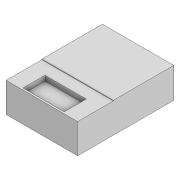
# Autodesk Inventor part: 00_HuaweiP30_Telelens
Saved by Autodesk Inventor 2022 (Build 260153000, 153)
## iProperties
Created: 2022-09-14
Part Number: 00_HuaweiP30_Telelens
Material: Generisch
Document SubType Name: Modeling
Designer: UC2
Density: 1 g/cm^3
Appearance: Vorgabe
Author: UC2
Autodesk Inventor part; units mm, degrees
ref_plane "YZ Plane" through (0, 0, 0) normal (1, 0, 0) x (0, 1, 0)
ref_plane "XZ Plane" through (0, 0, 0) normal (0, 1, 0) x (-1, 0, 0)
ref_plane "XY Plane" through (0, 0, 0) normal (0, 0, 1) x (1, 0, 0)
sketch "Skizze1" plane through (0, 0, 0) normal (0, 1, 0) x (-1, 0, 0)
  line L0 (-6.5, -8.75) -> (6.5, -8.75)
  line L1 (6.5, -8.75) -> (6.5, 8.75)
  line L2 (6.5, 8.75) -> (-6.5, 8.75)
  line L3 (-6.5, 8.75) -> (-6.5, -8.75)
  line L4 (-6.5, -8.75) -> (6.5, 8.75) construction
  line L5 (6.5, -8.75) -> (-6.5, 8.75) construction
  point P0 (0, 0)
  dimension "d0" = 13
  dimension "d1" = 17.5
  constraints: 12 end point, 2 midpoint, 2 parallel, 1 horizontal, 1 perpendicular
  measures "d0" distance of L2.end L1.end
  measures "d1" distance of L1.end L0.end
extrude "Extrusion1" add sketch "Skizze1" along normal blind 5.5
sketch "Skizze2" plane through (0, 5.5, 0) normal (0, 1, 0) x (1, 0, 0)
  line L0 (-6.5, 8.75) -> (-6.5, -8.75) projected
  line L1 (-6.5, -8.75) -> (6.5, -8.75) projected
  line L2 (6.5, -8.75) -> (6.5, 8.75) projected
  line L3 (6.5, 8.75) -> (-6.5, 8.75) projected
  line L4 (3.75, -4.4349) -> (-3.75, -4.4349)
  line L5 (-3.75, -4.4349) -> (-3.75, -8.4349)
  line L6 (-3.75, -8.4349) -> (3.75, -8.4349)
  line L7 (3.75, -8.4349) -> (3.75, -4.4349)
  line L8 (3.75, -4.4349) -> (-3.75, -8.4349) construction
  line L9 (-3.75, -4.4349) -> (3.75, -8.4349) construction
  point P0 (0, 0)
  point P1 (0, -6.4349)
  dimension "d4" = 7.5
  dimension "d5" = 4
  constraints: 12 end point, 2 midpoint, 2 parallel, 1 horizontal, 1 perpendicular
  measures "d4" distance of L6.end L5.end
  measures "d5" distance between parallel lines of L4 L6
extrude "Extrusion2" cut sketch "Skizze2" against normal blind 1 contours L7 L6 L5 L4
sketch "Skizze3" plane through (0, 5.5, 0) normal (0, 1, 0) x (1, 0, 0)
  line L0 (-6.5, 8.75) -> (-6.5, -8.75) projected
  line L1 (3.75, -8.4349) -> (-3.75, -8.4349) projected
  line L2 (-3.75, -8.4349) -> (-3.75, -4.4349) projected
  line L3 (-3.75, -4.4349) -> (3.75, -4.4349) projected
  line L4 (3.75, -4.4349) -> (3.75, -8.4349) projected
  line L5 (-6.5, 8.75) -> (-6.5, -8.75) projected
  line L6 (-6.5, -8.75) -> (6.5, -8.75) projected
  line L7 (6.5, -8.75) -> (6.5, 8.75) projected
  line L8 (6.5, 8.75) -> (-6.5, 8.75) projected
  line L9 (6.5, -8.75) -> (6.5, 8.75) projected
  line L10 (-6.5, -8.75) -> (6.5, -8.75)
  line L11 (6.5, -8.75) -> (6.5, -2.25)
  line L12 (6.5, -2.25) -> (-6.5, -2.25)
  line L13 (-6.5, -2.25) -> (-6.5, -8.75)
  point P0 (0, 0)
  dimension "d8" = 6.5
  constraints: 8 end point, 2 parallel, 1 horizontal, 1 perpendicular, 1 point on line
  measures "d8" distance of L11.end L10.end
extrude "Extrusion3" cut sketch "Skizze3" against normal blind 0.1 contours L12 L7 L6 L0
sketch "Skizze4" plane through (6.5, 0, -8.75) normal (0, 0, -1) x (-1, 0, 0)
  line L0 (0, 0) -> (13, 0) projected
  line L1 (13, 0) -> (13, 5.5) projected
  line L2 (0, 5.5) -> (13, 5.5) projected
  line L3 (0, 0) -> (0, 5.5) projected
  line L4 (10.15, 4.75) -> (2.85, 4.75)
  line L5 (2.85, 4.75) -> (2.85, 0.75)
  line L6 (2.85, 0.75) -> (10.15, 0.75)
  line L7 (10.15, 0.75) -> (10.15, 4.75)
  line L8 (10.15, 4.75) -> (2.85, 0.75) construction
  line L9 (2.85, 4.75) -> (10.15, 0.75) construction
  point P0 (6.5, 0)
  point P1 (6.5, 2.75)
  dimension "d11" = 7.3
  dimension "d12" = 4
  constraints: 12 end point, 2 midpoint, 2 parallel, 1 horizontal, 1 perpendicular
  measures "d11" distance of L6.end L5.end
  measures "d12" distance of L5.end L4.end
extrude "Extrusion4" cut sketch "Skizze4" against normal blind 0.1 contours L7 L6 L5 L4
